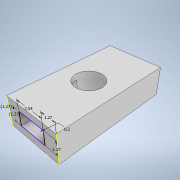
# Autodesk Inventor part: Block
Saved by Autodesk Inventor 2020.2 (Build 242310000, 310)
## iProperties
Created: 2020-04-17
Part Number: Block
Material: Generic
Document SubType Name: Modeling
Designer: Tanana
Density: 1 g/cm^3
Appearance: Default
Author: Tanana
Autodesk Inventor part; units mm, degrees
ref_plane "YZ Plane" through (0, 0, 0) normal (1, 0, 0) x (0, 1, 0)
ref_plane "XZ Plane" through (0, 0, 0) normal (0, 1, 0) x (-1, 0, 0)
ref_plane "XY Plane" through (0, 0, 0) normal (0, 0, 1) x (1, 0, 0)
sketch "Sketch1" plane through (0, 0, 0) normal (0, 1, 0) x (-1, 0, 0)
  line L0 (40.1367, 46.4954) -> (-10.6633, 46.4954)
  line L1 (-10.6633, 46.4954) -> (-10.6633, -55.1046)
  line L2 (-10.6633, -55.1046) -> (40.1367, -55.1046)
  line L3 (40.1367, -55.1046) -> (40.1367, 46.4954)
  circle A0 centre (14.7367, -4.3046) radius 12.7
  point P0 (0, 0)
  dimension "d0" = 101.6
  dimension "d1" = 50.8
  dimension "d21" = 25.4
  dimension "d22" = 50.8
  constraints: 8 end point, 2 parallel, 1 centre point, 1 horizontal, 1 perpendicular
  measures "d0" distance of L2.end L0.start
  measures "d1" distance of L0.start L0.end
  measures "d21" distance from line of L1 A0.centre
  measures "d22" distance from line of L0 A0.centre
extrude "Extrusion1" add sketch "Sketch1" along normal blind 25.4
sketch "Sketch2" plane through (-40.1367, 0, 46.4954) normal (0, 0, 1) x (1, 0, 0)
  line L0 (12.7, 19.8094) -> (36.1, 19.8094)
  line L1 (38.1, 17.8094) -> (38.1, 7.1094)
  line L2 (38.1, 7.1094) -> (12.7, 7.1094)
  line L3 (12.7, 7.1094) -> (12.7, 19.8094)
  line L4 (50.8, 0) -> (50.8, 25.4) projected
  line L5 (0, 0) -> (0, 25.4) projected
  arc A0 (38.1, 17.8094) -> (36.1, 19.8094) centre (36.1, 17.8094) ccw
  point P0 (40.1367, 0)
  point P1 (38.1, 19.8094)
  dimension "d5" = 25.4
  dimension "d6" = 12.7
  dimension "d7" = 12.7
  dimension "d8" = 12.7
  dimension "d9" = 12.7
  dimension "d10" = 2
  constraints: 8 end point, 2 parallel, 2 point on circle, 2 point on line, 2 tangent, 1 centre point, 1 horizontal, 1 perpendicular
  measures "d5" distance of L0.start point (38.1, 19.809)
  measures "d6" distance of point (38.1, 19.809) L1.end
  measures "d7" distance from line of L4 point (38.1, 19.809)
  measures "d8" distance between parallel lines of L5 L3
  measures "d9" distance of L2.end L0.start
  measures "d10" radius of A0
extrude "Extrusion2" cut sketch "Sketch2" against normal up to next
equation "\"d1\" = 0.5 * d0"
equation "\"d21\" = 0.5 * d1"
equation "\"d22\" = 0.5 * d0"
body "Solid1"
